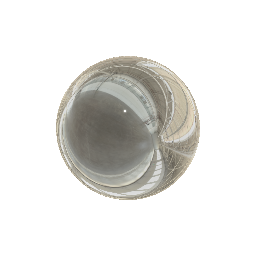
⅜” (9.52mm) Ball Bearing v2 (Autodesk Fusion 360 design; units mm, degrees)
Autodesk Fusion 360 part; units mm, degrees
sphere "SpherePrimitive1" add diameter 9.52 placed x (1, 0, 0) y (0, 1, 0) z (0, 0, 1) at (0, 0, 0)
